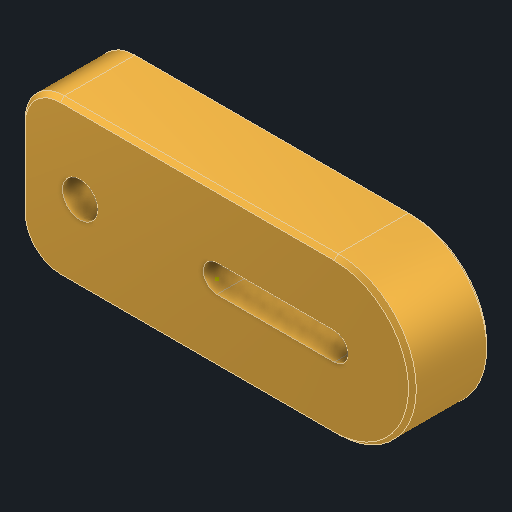
# Autodesk Inventor part: Bell Support Beam
Saved by Autodesk Inventor 2027.1 (Build 311270010, 270A)
## iProperties
Created: 2025-09-16
Material: Brass, Soft Yellow
Document SubType Name: Modeling
Designer: SD
Density: 8.47 g/cm^3
Appearance: Brass - Satin
Mass: 186.202 g
Surface Area: 68.7309 cm^2
Volume: 21.9837 cm^3
Project: Automatic Tea Steeping mechanism
Part Number: Bell Support Beam
Thickness: 10.000 mm
Length: 50.000 mm
Width: 20.000 mm
BOM-Mass: 0.18620
BOM-Area: 0.007
Procurement: Fabricate - 2nd round
Build Stage: 3
Preferred Material: C36000 Brass
Author: SD
Title: Bell Support Beam
Autodesk Inventor part; units mm, degrees
ref_plane "YZ Plane" through (0, 0, 0) normal (1, 0, 0) x (0, 1, 0)
ref_plane "XZ Plane" through (0, 0, 0) normal (0, 1, 0) x (-1, 0, 0)
ref_plane "XY Plane" through (0, 0, 0) normal (0, 0, 1) x (1, 0, 0)
sketch "Sketch1" plane through (0, 0, 0) normal (1, 0, 0) x (0, 1, 0)
  line L0 (-10, 5) -> (10, 5)
  line L1 (10, 5) -> (10, -5)
  line L2 (10, -5) -> (-10, -5)
  line L3 (-10, -5) -> (-10, 5)
  line L4 (-10, 5) -> (10, -5) construction
  line L5 (10, 5) -> (-10, -5) construction
  point P0 (0, 0)
  dimension "Width" = 20
  dimension "Thickness" = 10
  constraints: 12 end point, 2 midpoint, 2 parallel, 1 horizontal, 1 perpendicular
  measures "Width" distance of L1.end L2.end
  measures "Thickness" distance of L0.end L1.end
extrude "Extrusion1" add sketch "Sketch1" along normal mid plane 50
sketch "Sketch6" plane through (25, 10, -5) normal (0, 0, -1) x (-1, 0, 0)
  line L0 (50, 0) -> (50, -20) projected
  line L1 (50, 0) -> (0, 0) projected
  point P0 (25, -10)
  point P1 (42.5, -10)
  dimension "d40" = 7.5
  dimension "d56" = 10
  measures "d40" distance from line of point (42.5, -10) L0
  measures "d56" distance from line of point (42.5, -10) L1
hole "Hole5" at (-17.5, 0, -5) direction (0, 0, 1) diameter 4.5 depth 10.65 tip angle 118 countersink diameter 9.5 countersink angle 90
sketch "Sketch7" plane through (-25, -10, 5) normal (0, 0, 1) x (1, 0, 0)
  point P0 (25, 10)
fillet "Fillet1" radius 10 2 edges at (25, 10, 0) (25, -10, 0)
sketch "Sketch9" plane through (-25, -10, -5) normal (0, 0, -1) x (-1, 0, 0)
  line L0 (-25, 10) -> (-40, 10) construction
  line L1 (-25, 11.75) -> (-40, 11.75)
  line L2 (-40, 8.25) -> (-25, 8.25)
  arc A0 (-25, 8.25) -> (-25, 11.75) centre (-25, 10) ccw
  arc A1 (-40, 11.75) -> (-40, 8.25) centre (-40, 10) ccw
  line L3 (0, 20) -> (0, 0) projected
  line L4 (-40, 0) -> (0, 0) projected
  point P0 (-32.5, 10)
  dimension "d58" = 15
  dimension "d59" = 25
  dimension "d60" = 10
  dimension "d62" = 3.5
  constraints: 8 end point, 4 point on circle, 4 tangent, 2 centre point, 1 horizontal, 1 midpoint, 1 parallel
  measures "d58" distance of L0.end L0.start
  measures "d59" distance from line of L0.start L3
  measures "d60" distance from line of L0.start L4
  measures "d62" distance between parallel lines of L1 L2
extrude "Extrusion2" cut sketch "Sketch9" against normal blind 10
fillet "Fillet2" radius 5 2 edges at (-25, 10, 0) (-25, -10, 0)
chamfer "Chamfer1" distance 0.5 angle 45 16 edges at (-2.4999, 10, -5) (22.0711, -7.0711, -5) (25, 0, -5) (22.0711, 7.0711, -5) (-2.4999, -10, -5) (-23.5355, -8.5355, -5) (-25, 0, -5) (-23.5355, 8.5355, -5) (-2.4999, 10, 5) (22.0711, 7.0711, 5) (25, 0, 5) (22.0711, -7.0711, 5) (-2.4999, -10, 5) (-23.5355, -8.5355, 5) (-25, 0, 5) (-23.5355, 8.5355, 5)
body "Solid1"
